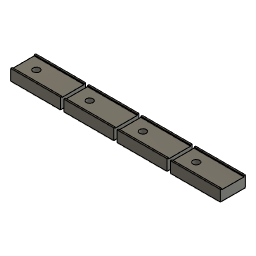
Rear Axle Support Spacer v3 (Autodesk Fusion 360 design; units mm, degrees)
Autodesk Fusion 360 part; units mm, degrees
sketch "Sketch1" plane through (0, 0, 0) normal (0, 1, 0) x (1, 0, 0)
  line L0 (0, 0) -> (48.26, 0)
  line L1 (48.26, 0) -> (48.26, -24.257)
  line L2 (48.26, -24.257) -> (0, -24.257)
  line L3 (0, -24.257) -> (0, 0)
  line L4 (0, -1.397) -> (48.26, -1.397)
  line L5 (48.26, -1.397) -> (48.26, -22.86)
  line L6 (48.26, -22.86) -> (0, -22.86)
  line L7 (0, -22.86) -> (0, -1.397)
  line L8 (0, -12.1285) -> (48.26, -12.1285) construction
  circle A0 centre (12.827, -12.1285) radius 3.175
  line L9 (0, -12.1285) -> (12.827, -12.1285)
  line L10 (51.562, -1.397) -> (99.822, -1.397)
  line L11 (51.562, 0) -> (99.822, 0)
  line L12 (99.822, -1.397) -> (99.822, -22.86)
  line L13 (51.562, -12.1285) -> (99.822, -12.1285) construction
  line L14 (99.822, -24.257) -> (51.562, -24.257)
  circle A1 centre (64.389, -12.1285) radius 3.175
  line L15 (99.822, -22.86) -> (51.562, -22.86)
  line L16 (51.562, -24.257) -> (51.562, 0)
  line L17 (51.562, -22.86) -> (51.562, -1.397)
  line L18 (99.822, 0) -> (99.822, -24.257)
  line L19 (51.562, -12.1285) -> (64.389, -12.1285)
  line L20 (-3.302, 0) -> (206.248, 0)
  line L21 (103.124, -1.397) -> (151.384, -1.397)
  line L22 (151.384, -1.397) -> (151.384, -22.86)
  line L23 (151.384, -24.257) -> (103.124, -24.257)
  line L24 (103.124, -22.86) -> (103.124, -1.397)
  line L25 (103.124, -12.1285) -> (115.951, -12.1285)
  circle A2 centre (115.951, -12.1285) radius 3.175
  line L26 (151.384, -22.86) -> (103.124, -22.86)
  line L27 (103.124, -12.1285) -> (151.384, -12.1285) construction
  line L28 (151.384, 0) -> (151.384, -24.257)
  line L29 (103.124, 0) -> (151.384, 0)
  line L30 (103.124, -24.257) -> (103.124, 0)
  line L31 (154.686, -1.397) -> (202.946, -1.397)
  line L32 (202.946, -1.397) -> (202.946, -22.86)
  line L33 (202.946, -24.257) -> (154.686, -24.257)
  line L34 (154.686, -22.86) -> (154.686, -1.397)
  line L35 (154.686, -12.1285) -> (167.513, -12.1285)
  circle A3 centre (167.513, -12.1285) radius 3.175
  line L36 (202.946, -22.86) -> (154.686, -22.86)
  line L37 (154.686, -12.1285) -> (202.946, -12.1285) construction
  line L38 (202.946, 0) -> (202.946, -24.257)
  line L39 (154.686, 0) -> (202.946, 0)
  line L40 (154.686, -24.257) -> (154.686, 0)
  line L41 (-3.302, 0) -> (206.248, 0)
  line L42 (206.248, 0) -> (206.248, -24.257)
  line L43 (206.248, -24.257) -> (-3.302, -24.257)
  line L44 (-3.302, -24.257) -> (-3.302, 0)
  point P0 (51.562, 0)
  point P1 (103.124, 0)
  point P2 (154.686, 0)
  dimension "d1" = 48.26
  dimension "d2" = 24.257
  dimension "d3" = 21.463
  dimension "d4" = 6.35
  dimension "d6" = 12.827
  dimension "d11" = 48.26
  dimension "d12" = 24.257
  dimension "d13" = 21.463
  dimension "d14" = 6.35
  dimension "d15" = 12.827
  dimension "d17" = 48.26
  dimension "d18" = 24.257
  dimension "d19" = 21.463
  dimension "d20" = 6.35
  dimension "d21" = 12.827
  dimension "d22" = 48.26
  dimension "d23" = 24.257
  dimension "d24" = 21.463
  dimension "d25" = 6.35
  dimension "d26" = 12.827
  dimension "d27" = 3.302
  dimension "d28" = 3.302
  dimension "d29" = 3.302
  dimension "d30" = 3.302
  dimension "d31" = 3.302
  dimension "d32" = 209.55
  dimension "d33" = 24.257
  constraint horizontal L0
  constraint vertical L1
  constraint horizontal L2
  constraint vertical L3
  constraint horizontal L4
  constraint vertical L5
  constraint horizontal L6
  constraint vertical L7
  constraint coincident L1 L5.end
  constraint coincident L3 L4.start
  constraint midpoint L3 L8.start
  constraint midpoint L1 L8.end
  constraint symmetric L4 L6 L8
  constraint coincident L8 A0.centre
  constraint perpendicular L7 L9
  constraint coincident A0.centre L9.end
  constraint horizontal L11
  constraint vertical L18
  constraint horizontal L14
  constraint vertical L16
  constraint coincident P0 L11.start
  constraint horizontal L10
  constraint vertical L12
  constraint horizontal L15
  constraint vertical L17
  constraint coincident L12.end L18
  constraint coincident L10.start L16
  constraint midpoint L13.start L16
  constraint midpoint L13.end L18
  constraint symmetric L10 L13 L15
  constraint coincident A1.centre L13
  constraint perpendicular L17 L19
  constraint coincident A1.centre L19.end
  constraint perpendicular L12 L20
  constraint horizontal L29
  constraint vertical L28
  constraint horizontal L23
  constraint vertical L30
  constraint coincident P1 L29.start
  constraint horizontal L21
  constraint vertical L22
  constraint horizontal L26
  constraint vertical L24
  constraint coincident L22.end L28
  constraint coincident L21.start L30
  constraint midpoint L25.start L30
  constraint midpoint L27.end L28
  constraint symmetric L21 L26 L27
  constraint coincident L25.end L27
  constraint perpendicular L24 L25
  constraint coincident L25.end A2.centre
  constraint horizontal L39
  constraint vertical L38
  constraint horizontal L33
  constraint vertical L40
  constraint coincident P2 L39.start
  constraint horizontal L31
  constraint vertical L32
  constraint horizontal L36
  constraint vertical L34
  constraint coincident L32.end L38
  constraint coincident L31.start L40
  constraint midpoint L35.start L40
  constraint midpoint L37.end L38
  constraint symmetric L31 L36 L37
  constraint coincident L35.end L37
  constraint perpendicular L34 L35
  constraint coincident L35.end A3.centre
  constraint coincident L0.start L20
  constraint horizontal L41
  constraint vertical L42
  constraint horizontal L43
  constraint vertical L44
  measures "d1" distance of L0.start L0.end
  measures "d2" distance of L0.end L1.end
  measures "d3" distance of L4 L6
  measures "d4" diameter of A0
  measures "d6" distance of L8.start A0.centre
  measures "d11" distance of L11.end P0
  measures "d12" distance of L11.end L14.start
  measures "d13" distance of L10 L15
  measures "d14" diameter of A1
  measures "d15" distance of A1.centre L13.start
  measures "d17" distance of L28.start P1
  measures "d18" distance of L23.start L28.start
  measures "d19" distance of L21 L26
  measures "d20" diameter of A2
  measures "d21" distance of L25.end L25.start
  measures "d22" distance of L38.start P2
  measures "d23" distance of L33.start L38.start
  measures "d24" distance of L31 L36
  measures "d25" diameter of A3
  measures "d26" distance of L35.end L35.start
  measures "d27" distance of L28 L34
  measures "d28" distance of L18 L30
  measures "d29" distance of L5 L16
  measures "d30" distance of L20.end L38
  measures "d31" distance of L0.start L20.start
  measures "d32" distance of L20.start L20.end
  measures "d33" distance of L20.start L43.end
extrude "Extrude1" add sketch "Sketch1" along normal blind 9.7028 contours L1 L3 L4 L5 L6 L7 | L10 L12 L15 L16 L17 L18 | L21 L22 L24 L26 L28 L30 | L31 L32 L34 L36 L38 L40 makes body 1 at (37.5073, 0, 12.1285) makes body 2 at (89.0693, 0, 12.1285) makes body 3 at (140.6313, 0, 12.1285) makes body 4 at (192.1933, 0, 12.1285)
extrude "Extrude2" add sketch "Sketch1" along normal blind 10.6934 contours L0 L1 L3 L4 L20 L41 | L10 L11 L16 L18 L20 L41 | L1 L2 L3 L6 L43 | L20 L21 L28 L29 L30 L41 | L14 L15 L16 L18 L43 | L20 L31 L38 L39 L40 L41 | L23 L26 L28 L30 L43 | L33 L36 L38 L40 L43 bodies 2 3 1 4
equation "d6 = 0.38 in + 0.125 in"
equation "d15 = 0.38 in + 0.125 in"
equation "d21 = 0.38 in + 0.125 in"
equation "d26 = 0.38 in + 0.125 in"
